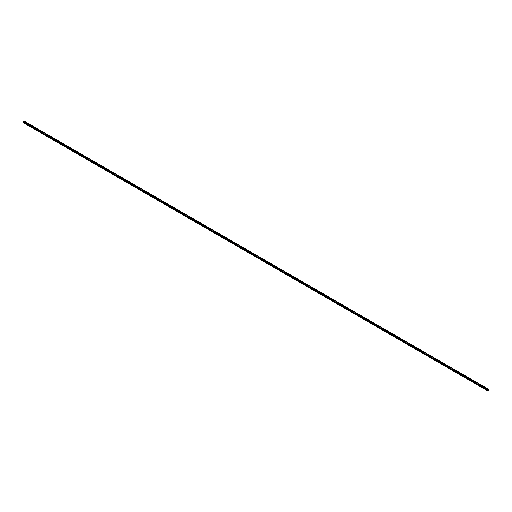
# Autodesk Inventor part: TL20240701-10100CV-RAIL 1
Saved by Autodesk Inventor 2022.5 (Build 265521000, 521)
## iProperties
Category: PROFILE ASSY
Manager: 호상태
Created: 2023-01-20
Part Number: TL20240701-10100CV-RAIL 1
User Status: 2
Material: SS400
Description: 3
Document SubType Name: Modeling
Designer: 박성규
Density: 7.85 g/cm^3
Appearance: 후처리 없음
DETAIL: Coveryor Assembly
M/C TITLE: CJ 제일제당 협동로봇 포장시스탬 PILOT 장비
PARTS NAME: Bracket
SPECIFICATION: TA20221101-CV200000-015
DocNumber: 221118_Standard_v1
Folder: .\
VDS_Category: 엔지니어링
Detail Description: Purchased products
Title: GUIDE A
Author: 박성규
Revision Number: A
Autodesk Inventor part; units mm, degrees
ref_plane "YZ Plane" through (0, 0, 0) normal (1, 0, 0) x (0, 1, 0)
ref_plane "XZ Plane" through (0, 0, 0) normal (0, 1, 0) x (-1, 0, 0)
ref_plane "XY Plane" through (0, 0, 0) normal (0, 0, 1) x (1, 0, 0)
sketch "스케치8" plane through (0, 0, 0) normal (1, 0, 0) x (0, 1, 0)
  line L0 (6, 8) -> (-6, 8)
  line L1 (-6, 8) -> (-6, -8)
  line L2 (-6, -8) -> (6, -8)
  line L3 (6, -8) -> (6, 8)
  line L4 (6, 8) -> (-6, -8) construction
  line L5 (-6, 8) -> (6, -8) construction
  point P0 (0, 0)
  dimension "d38" = 16
  dimension "d39" = 12
  constraints: 12 end point, 2 midpoint, 2 parallel, 1 horizontal, 1 perpendicular
  measures "d38" distance of L2.end L0.start
  measures "d39" distance of L1.end L2.end
extrude "돌출3" add sketch "스케치8" along normal mid plane 7680
sketch "스케치9" plane through (-3840, 6, 8) normal (0, 1, 0) x (1, 0, 0)
  line L0 (0, 16) -> (7680, 16) construction
  line L1 (7680, 16) -> (7680, 0) construction
  line L2 (0, 16) -> (7680, 16) projected
  line L3 (3840, 16) -> (3840, 0) construction
  line L4 (0, 0) -> (7680, 0) projected
  point P0 (3840, 8)
  point P1 (7660, 8)
  point P2 (20, 8)
  dimension "d42" = 8
  dimension "d43" = 20
  constraints: 2 end point, 2 midpoint, 1 symmetric about line
  measures "d42" distance from line of L0 point (7660, 8)
  measures "d43" distance from line of L1 point (7660, 8)
hole "구멍3" at (3820, 6, 0) at (-3820, 6, 0) direction (0, -1, 0) diameter 6.6 end through all counterbore diameter 11 counterbore depth 6.8 clearance for "Socket Head Cap Screw ISO 4762" size "M6" standard "ISO"
chamfer "Chamfer1" distance 5 distance2 15 1 edges at (-3840, 0, -8) measured on face at (-3840, 0, -7.5)
chamfer "Chamfer2" distance 5 distance2 15 1 edges at (3840, 0, -8) measured on face at (3840, 0, -7.5)
equation "\"d40\" = L1 + L2"
equation "\"L1\" = 6000"
equation "\"L2\" = 1680"
